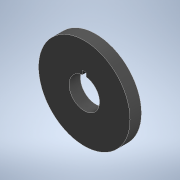
# Autodesk Inventor part: clutch03-simplyGearDisk
Saved by Autodesk Inventor 2021 (Build 250183000, 183)
## iProperties
Created: 2020-07-03
Part Number: clutch03-simplyGearDisk
Material: Polycarbonate, Smoke
Document SubType Name: Modeling
Designer: robst
Density: 1.2 g/cm^3
Appearance: Generic
Author: robst
Autodesk Inventor part; units mm, degrees
ref_plane "YZ Plane" through (0, 0, 0) normal (1, 0, 0) x (0, 1, 0)
ref_plane "XZ Plane" through (0, 0, 0) normal (0, 1, 0) x (-1, 0, 0)
ref_plane "XY Plane" through (0, 0, 0) normal (0, 0, 1) x (1, 0, 0)
sketch "Sketch5" plane through (0, 0, 0) normal (0, 0, 1) x (1, 0, 0)
  circle A0 centre (0, 0) radius 38.1
  circle A1 centre (0, 0) radius 12.7
  arc A2 (1.5875, 15.7954) -> (-1.5875, 15.7954) centre (0, 0) ccw
  line L0 (0, 0) -> (0, 15.875) construction
  line L1 (-1.5875, 15.7954) -> (-1.5875, 12.6004)
  line L2 (1.5875, 12.6004) -> (1.5875, 15.7954)
  dimension "d11" = 76.2
  dimension "d12" = 25.4
  dimension "d13" = 31.75
  dimension "d14" = 1.5875
  dimension "d15" = 1.5875
  constraints: 6 end point, 5 point on circle, 3 centre point, 3 coincident, 2 parallel, 1 vertical
  measures "d11" diameter of A0
  measures "d12" diameter of A1
  measures "d13" diameter of A2
  measures "d14" distance between parallel lines of L1 L0
  measures "d15" distance between parallel lines of L0 L2
extrude "Extrusion4" add sketch "Sketch5" along normal blind 9.525
body "Solid2"
